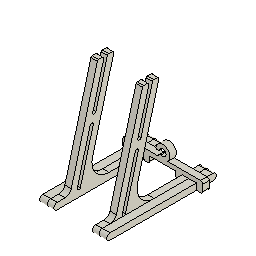
LCA Badge Stand v3.1 (Autodesk Fusion 360 design; units mm, degrees)
Autodesk Fusion 360 part; units mm, degrees
note: some values were not read from the file. Chosen so that the rebuilt part matches the saved one: which face or edge a step refers to. Set by a fixed rule: which sketch regions a step uses.
sketch "Sketch1" plane through (0, 0, 0) normal (1, 0, 0) x (0, 1, 0)
  circle A0 centre (-67.0553, 26.6271) radius 2.5
  line L0 (-67.0553, 29.1271) -> (12.9447, 29.1271)
  line L1 (12.9447, 29.1271) -> (12.9447, 24.1271)
  line L2 (12.9447, 24.1271) -> (-67.0553, 24.1271)
  line L3 (-67.0553, 24.1271) -> (-67.0553, 29.1271)
  circle A1 centre (12.9447, 26.6271) radius 2.5
  line L4 (-57.0553, 29.1271) -> (-57.0553, 44.2726) construction
  line L5 (-57.0553, 29.1271) -> (-35.818, 108.3859)
  line L6 (-34.8521, 109.1271) -> (-31.7462, 109.1271)
  line L7 (-30.7803, 107.8682) -> (-51.8789, 29.1271)
  line L8 (-49.2908, 29.1271) -> (-28.0534, 108.3859)
  line L9 (-23.0157, 107.8682) -> (-44.1144, 29.1271)
  line L10 (-27.0875, 109.1271) -> (-23.9817, 109.1271)
  arc A2 (-34.8521, 109.1271) -> (-35.818, 108.3859) centre (-34.8521, 108.1271) ccw
  arc A3 (-30.7803, 107.8682) -> (-31.7462, 109.1271) centre (-31.7462, 108.1271) ccw
  arc A4 (-27.0875, 109.1271) -> (-28.0534, 108.3859) centre (-27.0875, 108.1271) ccw
  arc A5 (-23.0157, 107.8682) -> (-23.9817, 109.1271) centre (-23.9817, 108.1271) ccw
  line L11 (-37.233, 74.1271) -> (-39.8212, 74.1271)
  line L12 (-41.161, 69.1271) -> (-38.5728, 69.1271)
  circle A6 centre (-40.2305, 67.855) radius 1.272
  circle A7 centre (-38.1922, 75.3771) radius 1.25
  line L13 (-38.1922, 75.3771) -> (-39.4422, 75.3771)
  line L14 (-38.1922, 75.3771) -> (-36.9422, 75.3771)
  line L15 (-40.2305, 67.855) -> (-41.5025, 67.8524)
  line L16 (-40.2305, 67.855) -> (-38.9585, 67.8577)
  circle A8 centre (-50.2499, 30.3771) radius 1.25
  dimension "d6" = 5
  dimension "d7" = 80
  dimension "d8" = 5
  dimension "d9" = 10
  dimension "d10" = 2.5
  dimension "d11" = 5
  dimension "d12" = 5
  dimension "d13" = 75
  dimension "d16" = 1
  dimension "d17" = 1
  dimension "d18" = 1
  dimension "d19" = 1
  dimension "d20" = 80
  dimension "d35" = 5
  dimension "d36" = 35
  constraint horizontal L0
  constraint vertical L1
  constraint horizontal L2
  constraint vertical L3
  constraint coincident A0.centre L3
  constraint tangent A0 L0
  constraint tangent A0 L2
  constraint midpoint L1 A1.centre
  constraint coincident L0 L4.start
  constraint perpendicular L0 L4
  constraint perpendicular L4 L6
  constraint parallel L5 L7
  constraint coincident L0 L7.end
  constraint parallel L8 L9
  constraint coincident L0 L8.start
  constraint coincident L0 L9.end
  constraint collinear L6 L10
  constraint tangent L5 A2
  constraint tangent L6 A2
  constraint tangent L6 A3
  constraint tangent L7 A3
  constraint tangent L8 A4
  constraint tangent L10 A4
  constraint tangent L9 A5
  constraint tangent L10 A5
  constraint coincident L8 L11.start
  constraint coincident L7 L11.end
  constraint horizontal L11
  constraint coincident L7 L12.start
  constraint coincident L8 L12.end
  constraint parallel L11 L12
  constraint tangent L12 A6
  constraint tangent L8 A6
  constraint tangent L11 A7
  constraint tangent L7 A7
  constraint tangent L8 A7
  constraint coincident A7.centre L13.start
  constraint coincident A7 L13.end
  constraint horizontal L13
  constraint coincident A7 L14.end
  constraint parallel L13 L14
  constraint coincident A6.centre L15.start
  constraint coincident A6 L15.end
  constraint coincident L7 L15.end
  constraint coincident A6 L16.end
  constraint parallel L15 L16
  constraint tangent L0 A8
  constraint tangent L7 A8
  constraint tangent L8 A8
  measures "d6" diameter of A0
  measures "d7" distance of L0.start L1
  measures "d8" diameter of A1
  measures "d9" distance of L0.start L4
  measures "d10" distance of L7 L8
  measures "d11" distance of L5 L7
  measures "d12" distance of L8 L9
  measures "d13" angle of L0 L7
  measures "d16" radius of A2
  measures "d17" radius of A3
  measures "d18" radius of A4
  measures "d19" radius of A5
  measures "d20" distance of L0 L6
  measures "d35" distance of L11 L12
  measures "d36" distance of L6 L11
extrude "Extrude1" add sketch "Sketch1" along normal blind 5 contours A0 L3 | A0 L0 L2 A1 | A0 L3 | L0 L5 L6 L7 A2 A3 A6 | L1 A1 | L1 A1 | L0 L7 A8 | L0 L8 A8 | L0 L8 L9 L10 A4 A5 | L7 A6 | L8 L12 A6 | L7 L12 A6 | L7 L8 L11 L12 | L7 L11 A7 | L8 L11 A7 makes body 1
fillet "FrontFillet" radius 5 1 edges at (2.5, -57.0553, 29.1271) on bodies 1
fillet "RearArmFillet" radius 13.3333 1 edges at (2.5, -44.1144, 29.1271) on bodies 1
extrude "AddBaseThickener" add sketch "Sketch1" against normal blind 6 separate body contours A0 L3 | A0 L0 L2 A1 | A0 L3 | L1 A1 | L1 A1 makes body 2
copy_body "CutPasteBodies2" bodies 1 2 removing the originals makes body 3 makes body 4 in component "LeftArm (original)"
ref_plane "WorkPlane1" through (20, -27.0553, 66.6271) normal (1, 0, 0) x (0, 1, 0)
mirror "MirrorComponent1" about plane through (0, 0, 0) normal (0, 0, 1) of bodies 3 4 makes body 5 at (5, -26.9496, -25.7937) makes body 6 at (-2, -13.722, -24.1271) in component "RightArm"
sketch "Sketch2" plane through (0, 0, 29.1271) normal (0, 0, 1) x (-1, 0, 0) in component "USBCableHolder"
  line L0 (-35, 26.738) -> (-40, 26.738)
  line L1 (-40, 26.738) -> (-40, -12.9447)
  line L2 (-40, -12.9447) -> (-35, -12.9447)
  line L3 (-35, -12.9447) -> (-35, 26.738)
  line L4 (-40, -12.9447) -> (-40, 67.0553)
  line L5 (-40, 67.0553) -> (-46, 67.0553)
  line L6 (-46, 67.0553) -> (-46, -12.9447)
  line L7 (-46, -12.9447) -> (-40, -12.9447)
  line L8 (0, 67.0553) -> (0, -12.9447)
  line L9 (0, -12.9447) -> (6, -12.9447)
  line L10 (6, -12.9447) -> (6, 67.0553)
  line L11 (6, 67.0553) -> (0, 67.0553)
  line L12 (0, 26.738) -> (-5, 26.738)
  line L13 (-5, 26.738) -> (-5, -12.9447)
  line L14 (-5, -12.9447) -> (0, -12.9447)
  line L15 (0, -12.9447) -> (0, 26.738)
  line L16 (-20, 78.0553) -> (-20, -23.9447)
  line L17 (-35, -12.9447) -> (-5, -12.9447) construction
  line L18 (-35, 2.0553) -> (-5, 2.0553) construction
  dimension "d49" = 15
  constraint coincident L2.end L3.start
  constraint coincident L13.end L14.start
  constraint coincident L3 L18.start
  constraint coincident L13 L18.end
  constraint perpendicular L13 L18
  measures "d49" distance of L17 L18
sketch "Sketch3" plane through (0, 0, 0) normal (0, 1, 0) x (1, 0, 0) in component "USBCableHolder"
  line L0 (46, -29.1271) -> (51, -29.1271)
  line L1 (51, -29.1271) -> (51, -30.7937)
  line L2 (49.3333, -32.4604) -> (46, -32.4604)
  line L3 (46, -32.4604) -> (46, -29.1271)
  line L4 (35, -29.1271) -> (5, -29.1271)
  line L5 (20, -29.1271) -> (20, -29.773)
  line L6 (20, -29.773) -> (20, -49.5969) construction
  line L7 (46, -32.4604) -> (20, -32.4604)
  line L8 (35, -29.1271) -> (20, -29.1271)
  line L9 (46, -29.1271) -> (35, -29.1271)
  arc A0 (49.3333, -32.4604) -> (51, -30.7937) centre (49.3333, -30.7937) ccw
  line L10 (51, -29.1271) -> (46, -29.1271)
  line L11 (46, -29.1271) -> (46, -25.7937)
  line L12 (47.6667, -24.1271) -> (49.3333, -24.1271)
  line L13 (51, -25.7937) -> (51, -29.1271)
  arc A1 (51, -25.7937) -> (49.3333, -24.1271) centre (49.3333, -25.7937) ccw
  arc A2 (47.6667, -24.1271) -> (46, -25.7937) centre (47.6667, -25.7937) ccw
  line L14 (46, -32.4604) -> (20, -32.4604)
  line L15 (20, -32.4604) -> (20, -29.1271)
  line L16 (20, -29.1271) -> (46, -29.1271)
  line L17 (46, -29.1271) -> (46, -32.4604)
  circle A3 centre (20, -36.4604) radius 2.5
  circle A4 centre (20, -36.4604) radius 5.5
  line L18 (35, -29.1271) -> (30, -29.1271)
  line L19 (30, -29.1271) -> (30, -25.7937)
  line L20 (31.6667, -24.1271) -> (33.3333, -24.1271)
  line L21 (35, -25.7937) -> (35, -29.1271)
  line L22 (40, -24.1271) -> (35, -24.1271)
  arc A5 (31.6667, -24.1271) -> (30, -25.7937) centre (31.6667, -25.7937) ccw
  arc A6 (35, -25.7937) -> (33.3333, -24.1271) centre (33.3333, -25.7937) ccw
  line L23 (-6, -32.4604) -> (20, -32.4604)
  line L24 (20, -29.1271) -> (-6, -29.1271)
  line L25 (5, -25.7937) -> (5, -29.1271)
  arc A7 (6.6667, -24.1271) -> (5, -25.7937) centre (6.6667, -25.7937) ccw
  arc A8 (10, -25.7937) -> (8.3333, -24.1271) centre (8.3333, -25.7937) ccw
  line L26 (10, -29.1271) -> (10, -25.7937)
  line L27 (8.3333, -24.1271) -> (6.6667, -24.1271)
  line L28 (-7.6667, -24.1271) -> (-9.3333, -24.1271)
  arc A9 (-6, -25.7937) -> (-7.6667, -24.1271) centre (-7.6667, -25.7937) ccw
  line L29 (-6, -29.1271) -> (-6, -25.7937)
  line L30 (-11, -25.7937) -> (-11, -29.1271)
  arc A10 (-11, -30.7937) -> (-9.3333, -32.4604) centre (-9.3333, -30.7937) ccw
  line L31 (-11, -29.1271) -> (-11, -30.7937)
  line L32 (-9.3333, -32.4604) -> (-6, -32.4604)
  arc A11 (-9.3333, -24.1271) -> (-11, -25.7937) centre (-9.3333, -25.7937) ccw
  line L33 (20, -36.4604) -> (14.5, -36.4604)
  line L34 (20, -36.4604) -> (16.1109, -32.5713)
  line L35 (20, -36.4604) -> (14.5688, -37.3276)
  line L36 (14.5688, -37.3276) -> (16.1109, -32.5713) construction
  line L37 (14.5688, -37.3276) -> (11.5688, -37.8065)
  line L38 (11.5688, -37.8065) -> (16, -32.4604)
  line L39 (16.1109, -32.5713) -> (16, -32.4604)
  line L40 (16, -32.4604) -> (13.0707, -32.4604) construction
  line L41 (11.5688, -37.8065) -> (11.6837, -32.4604) construction
  point P0 (46, -29.1271)
  point P1 (20, -29.1271)
  point P2 (46, -24.1271)
  dimension "d50" = 5
  dimension "d51" = 3.3333
  dimension "d52" = 1.6667
  dimension "d53" = 1.6667
  dimension "d54" = 1.6667
  dimension "d57" = 5
  dimension "d58" = 3
  dimension "d59" = 4
  dimension "d60" = 5
  dimension "d61" = 5
  dimension "d62" = 1.6667
  dimension "d63" = 1.6667
  dimension "d64" = 45
  dimension "d66" = 5
  dimension "d67" = 3
  constraint horizontal L0
  constraint vertical L1
  constraint horizontal L2
  constraint vertical L3
  constraint coincident P0 L0.start
  constraint coincident P1 L5.start
  constraint perpendicular L4 L5
  constraint perpendicular L4 L6
  constraint coincident L6 L7.end
  constraint perpendicular L6 L7
  constraint coincident L4.start L8.start
  constraint tangent L1 A0
  constraint tangent L2 A0
  constraint horizontal L10
  constraint vertical L11
  constraint horizontal L12
  constraint vertical L13
  constraint tangent L12 A1
  constraint tangent L13 A1
  constraint tangent L11 A2
  constraint tangent L12 A2
  constraint horizontal L14
  constraint vertical L15
  constraint horizontal L16
  constraint vertical L17
  constraint coincident L6 A3.centre
  constraint collinear L3 L11
  constraint horizontal L18
  constraint vertical L19
  constraint horizontal L20
  constraint vertical L21
  constraint collinear L20 L22
  constraint tangent L19 A5
  constraint tangent L20 A5
  constraint tangent L20 A6
  constraint tangent L21 A6
  constraint symmetric L0.end L6 L30.end
  constraint symmetric L2.end L6 L23.start
  constraint symmetric P1 L6 L5.start
  constraint symmetric L6 L7.end L14.end
  constraint symmetric L6 L1.end A10.start
  constraint symmetric L6 L2.start A10.end
  constraint symmetric L6 A0 A10
  constraint symmetric L6 P0 L24.end
  constraint symmetric L6 L12.end L28.end
  constraint symmetric L6 L13.start L30.start
  constraint symmetric L6 A1 A11
  constraint symmetric L6 L11.end A9.start
  constraint symmetric L6 L12.start L28.start
  constraint symmetric L6 A2 A9
  constraint symmetric L6 L4.start L4.end
  constraint symmetric L6 L18.end L26.start
  constraint symmetric L6 L19.end A8.start
  constraint symmetric L6 L20.start A8.end
  constraint symmetric L6 A5 A8
  constraint symmetric L6 L20.end A7.start
  constraint symmetric L6 L21.start L25.start
  constraint symmetric L6 A6 A7
  constraint coincident A3.centre A4.centre
  constraint coincident A4 L33.end
  constraint perpendicular L6 L33
  constraint coincident A4 L34.end
  constraint coincident A4 L35.end
  constraint parallel L35 L37
  constraint parallel L34 L39
  constraint coincident L23 L38.end
  constraint coincident L23 L40.end
  constraint coincident L23 L41.end
  measures "d50" distance of P0 L0.end
  measures "d51" distance of P0 L2.end
  measures "d52" radius of A0
  measures "d53" radius of A1
  measures "d54" radius of A2
  measures "d57" diameter of A3
  measures "d59" distance of L7 A3.centre
  measures "d60" distance of L0 L12
  measures "d61" distance of L19 L21
  measures "d62" radius of A5
  measures "d63" radius of A6
  measures "d64" angle of L33 L34
  measures "d66" distance of L34.end L35.end
  measures "d67" horizontal distance of L35.end L37.end
extrude "Extrude2" add sketch "Sketch3" along normal blind 5 separate body contours L0 L10 L11 L12 L13 A1 A2 | L0 L1 L2 L3 A0 L10 L17 | L3 L4 L5 L7 L8 L9 L14 L15 L16 L17 A4 L18 | L4 L8 L16 L18 L19 L20 L21 A5 A6 | L7 L14 A3 A4 L23 L34 L35 | L7 L14 L15 A4 | L15 A4 L23 | L4 L5 L15 A4 L23 L24 L28 A9 L29 L30 A10 L31 L32 A11 | A4 L23 L39 | A3 A4 L33 L35 | L4 L24 L25 A7 A8 L26 L27 makes body 7 in component "USBCableHolder"
fillet "Fillet2" radius 0.75 1 edges at (18.2322, 2.5, 34.6926) on bodies 7 in component "USBCableHolder"
fillet "Fillet4" radius 0.75 2 edges at (14.5, 2.5, 36.4604) (17.5, 2.5, 36.4604) on bodies 7 in component "USBCableHolder"
fillet "Fillet5" radius 0.75 1 edges at (16, 2.5, 32.4604) on bodies 7 in component "USBCableHolder"
component "LeftArm (original)" placed x (1, 0, 0) y (0, 1, 0) z (0, 0, 1) at (0, 0, 0)
component "RightArm" placed x (-1, 0, 0) y (0, 1, 0) z (0, 0, -1) at (40, 0, 0)
component "USBCableHolder" placed x (1, 0, 0) y (0, 1, 0) z (0, 0, 1) at (0, 0, 0)
equation "boardthickness = 2.5 mm"
equation "fillet = 1 mm"
equation "basethickness = 5 mm"
equation "baselength = 80 mm" comment "how long the base is"
equation "base_setback = 10 mm" comment "how far back from the front radius the arms are"
equation "d6 = basethickness"
equation "d7 = baselength"
equation "d8 = d6"
equation "d9 = base_setback"
equation "d10 = boardthickness"
equation "d11 = basethickness"
equation "d12 = d11"
equation "d13 = board_angle"
equation "board_angle = 75 deg"
equation "d16 = fillet"
equation "d17 = fillet"
equation "d20 = holderheight"
equation "holderheight = 80 mm" comment "how tall the arms are"
equation "d25 = basethickness"
equation "d27 = holderheight / 6"
equation "d28 = -thickener"
equation "thickener = 6 mm" comment "the extra width added to the feet"
equation "d35 = basethickness"
equation "d36 = topBadgeSpace"
equation "topBadgeSpace = 35 mm" comment "The depth of the slot in the top to hold the badge"
equation "legspacing = 30 mm" comment "the space between the legs"
equation "d40 = legspacing / 2"
equation "d49 = basethickness * 3"
equation "d50 = basethickness"
equation "d51 = basethickness * ( 2 / 3 )"
equation "d52 = basethickness / 3"
equation "d53 = basethickness / 3"
equation "d54 = basethickness / 3"
equation "USB_Cable_Thickness = 5 mm"
equation "USB_Cable_Holder_Offset = 3 mm"
equation "d57 = USB_Cable_Thickness"
equation "d58 = USB_Cable_Holder_Offset"
equation "d59 = ( USB_Cable_Thickness / 2 ) + ( USB_Cable_Holder_Offset / 2 )"
equation "d60 = basethickness"
equation "d61 = basethickness"
equation "d62 = basethickness / 3"
equation "d63 = basethickness / 3"
equation "d66 = USB_Cable_Thickness"
equation "d67 = USB_Cable_Holder_Offset"
equation "d68 = basethickness"
equation "d73 = USB_Cable_Holder_Offset / 4"
equation "d77 = USB_Cable_Holder_Offset / 4"
equation "d79 = USB_Cable_Holder_Offset / 4"
named bodies: "MainBit", "Thicker_Base"
